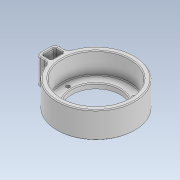
# Autodesk Inventor part: front_hip_mask
Saved by Autodesk Inventor 2020 (Build 240168000, 168)
## iProperties
Created: 2021-02-08
Part Number: front_hip_mask
Material: Generic
Document SubType Name: Modeling
Designer: DELL
Density: 1 g/cm^3
Appearance: Default
Author: DELL
Autodesk Inventor part; units mm, degrees
ref_plane "YZ Plane" through (0, 0, 0) normal (1, 0, 0) x (0, 1, 0)
ref_plane "XZ Plane" through (0, 0, 0) normal (0, 1, 0) x (-1, 0, 0)
ref_plane "XY Plane" through (0, 0, 0) normal (0, 0, 1) x (1, 0, 0)
sketch "Sketch1" plane through (0, 0, 0) normal (0, 1, 0) x (-1, 0, 0)
  circle A0 centre (0, 0) radius 46
  circle A1 centre (0, 0) radius 40
  circle A2 centre (0, 0) radius 28.5
  circle A3 centre (0, 0) radius 33 construction
  line L0 (0, 0) -> (16.5, 28.5788) construction
  line L1 (46, 0) -> (-46, 0) construction
  circle A4 centre (33, 0) radius 2.25
  circle A5 centre (16.5, 28.5788) radius 2.25
  circle A6 centre (33, 0) radius 3.75
  circle A7 centre (16.5, 28.5788) radius 3.75
  line L2 (0, 46) -> (0, -46) construction
  circle A8 centre (16.5, -28.5788) radius 2.25
  circle A9 centre (16.5, -28.5788) radius 3.75
  circle A10 centre (-16.5, 28.5788) radius 2.25
  circle A11 centre (-16.5, 28.5788) radius 3.75
  circle A12 centre (-16.5, -28.5788) radius 3.75
  circle A13 centre (-16.5, -28.5788) radius 2.25
  line L3 (0, 0) -> (-16.5, 28.5788) construction
  line L4 (-20, 34.641) -> (-0.3277, 45.9988)
  line L5 (-16.5, 28.5788) -> (-20, 34.641) construction
  line L6 (-20, -34.641) -> (-0.3277, -45.9988)
  line L7 (45.3845, 7.5) -> (56, 7.5)
  line L8 (56, 7.5) -> (56, -7.5)
  line L9 (56, -7.5) -> (45.3845, -7.5)
  line L10 (44.5393, -11.5) -> (60, -11.5)
  line L11 (60, -11.5) -> (60, 11.5)
  line L12 (60, 11.5) -> (44.5393, 11.5)
  line L13 (45.3845, -7.5) -> (45.3845, 7.5)
  dimension "d0" = 92
  dimension "d1" = 80
  dimension "d2" = 57
  dimension "d3" = 66
  dimension "d4" = 60
  dimension "d5" = 4.5
  dimension "d6" = 7.5
  dimension "d16" = 15
  dimension "d17" = 56
  dimension "d18" = 4
  dimension "d21" = 10
  constraints: 28 end point, 13 centre point, 10 coincident, 8 symmetric about line, 4 point on circle, 3 horizontal, 3 midpoint, 2 equal radius, 2 perpendicular, 2 point on line, 2 vertical, 1 collinear, 1 tangent, 21 other
  measures "d1" diameter of A1
  measures "d2" diameter of A2
  measures "d3" diameter of A3
  measures "d4" angle of L1 L0
  measures "d5" diameter of A4
  measures "d6" diameter of A6
  measures "d16" distance between parallel lines of L7 L9
  measures "d17" distance from line of point (0, 0) L8
  measures "d18" distance between parallel lines of L11 L8
  measures "d21" distance from line of L1.start L8
extrude "Extrusion1" add sketch "Sketch1" along normal blind 6 contours L13 A0 L6 A1 L4 | L4 A1 L6 A0 | A1 | A5 | A6 | A7 | A8 | A9 | A11 | A12
extrude "Extrusion2" add sketch "Sketch1" along normal blind 25 from surface at 6 contours L13 A0 L6 A1 L4 | L4 A1 L6 A0
extrude "Extrusion3" cut sketch "Sketch1" along normal blind 3 contours A4 | A6 | A10 | A11 | A12 | A13
fillet "Fillet1" [suppressed]
fillet "Fillet2" [suppressed]
extrude "Extrusion5" add sketch "Sketch1" along normal up to surface (31 mm away) contours A0 L12 L11 L10 L9 L8 L7
fillet "Fillet4" radius 6 4 edges at (-44.5393, 15.5, 11.5) (-44.5393, 15.5, -11.5) (-60, 15.5, -11.5) (-60, 15.5, 11.5)
fillet "Fillet5" radius 2 4 edges at (-45.3845, 15.5, -7.5) (-56, 15.5, -7.5) (-56, 15.5, 7.5) (-45.3845, 15.5, 7.5)
fillet "Fillet3" radius 1 21 edges at (-20, 6, 34.641) (46, 31, 0) (-20, 31, 34.641) (46, 0, 0) (28.5, 6, 0) (-55.4142, 31, -6.9142) (-56, 31, 0) (-55.4142, 31, 6.9142) (-50.6922, 31, 7.5) (-45.9703, 31, 6.9142) (-45.3845, 31, 0) (-45.9703, 31, -6.9142) (-50.6922, 31, -7.5) (-45.9703, 0, 6.9142) (-50.6922, 0, 7.5) (-55.4142, 0, 6.9142) (-56, 0, 0) (-55.4142, 0, -6.9142) (-50.6922, 0, -7.5) (-45.9703, 0, -6.9142) (-45.3845, 0, 0)
body "Solid1"
